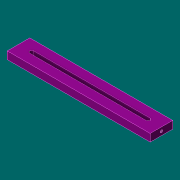
# Autodesk Inventor part: verticalSupourt
Saved by Autodesk Inventor 2016 (Build 200138000, 138)
## iProperties
Created: 2015-10-27
Part Number: verticalSupourt
Material: ABS Plastic
Document SubType Name: Modeling
Designer: Sawaiz
Density: 1.06 g/cm^3
Appearance: Smooth - Purple
Author: Sawaiz
Autodesk Inventor part; units mm, degrees
ref_plane "YZ Plane" through (0, 0, 0) normal (1, 0, 0) x (0, 1, 0)
ref_plane "XZ Plane" through (0, 0, 0) normal (0, 1, 0) x (-1, 0, 0)
ref_plane "XY Plane" through (0, 0, 0) normal (0, 0, 1) x (1, 0, 0)
sketch "Sketch1" plane through (0, 0, 0) normal (0, 0, 1) x (1, 0, 0)
  line L0 (-9.525, -60.325) -> (9.525, -60.325)
  line L1 (9.525, -60.325) -> (9.525, 60.325)
  line L2 (9.525, 60.325) -> (-9.525, 60.325)
  line L3 (-9.525, 60.325) -> (-9.525, -60.325)
  line L4 (-9.525, -60.325) -> (9.525, 60.325) construction
  line L5 (9.525, -60.325) -> (-9.525, 60.325) construction
  point P0 (0, 0)
  dimension "d0" = 19.05
  dimension "d1" = 120.65
  constraints: 12 end point, 2 midpoint, 2 parallel, 1 horizontal, 1 perpendicular
  measures "d0" distance of L2.end L1.end
  measures "d1" distance of L1.end L0.end
extrude "Extrusion1" add sketch "Sketch1" along normal blind 6.35
sketch "Sketch2" plane through (0, 0, 6.35) normal (0, 0, 1) x (1, 0, 0)
  line L0 (1.6891, -50.8) -> (-1.6891, -50.8)
  line L1 (-1.6891, -50.8) -> (-1.6891, 50.8)
  line L2 (-1.6891, 50.8) -> (1.6891, 50.8)
  line L3 (1.6891, 50.8) -> (1.6891, -50.8)
  line L4 (1.6891, -50.8) -> (-1.6891, 50.8) construction
  line L5 (-1.6891, -50.8) -> (1.6891, 50.8) construction
  point P0 (0, 0)
  dimension "d4" = 3.3782
  dimension "d5" = 101.6
  constraints: 12 end point, 2 midpoint, 2 parallel, 1 horizontal, 1 perpendicular
  measures "d4" distance of L1.end L2.end
  measures "d5" distance of L0.end L1.end
extrude "Extrusion2" cut sketch "Sketch2" against normal through all
fillet "Fillet1" radius 1.6891 4 edges at (-1.6891, -50.8, 3.175) (1.6891, -50.8, 3.175) (-1.6891, 50.8, 3.175) (1.6891, 50.8, 3.175)
sketch "Sketch4" plane through (-9.525, -60.325, 0) normal (0, -1, 0) x (1, 0, 0)
  line L0 (0, 0) -> (19.05, 0) projected
  line L1 (19.05, 0) -> (19.05, 6.35) projected
  line L2 (0, 6.35) -> (19.05, 6.35) projected
  line L3 (0, 0) -> (0, 6.35) projected
  point P0 (9.525, 0)
  point P1 (9.525, 3.175)
  dimension "d16" = 3.175
  dimension "d17" = 9.525
  measures "d16" distance from line of L0 point (9.525, 3.175)
  measures "d17" distance from line of L3 point (9.525, 3.175)
hole "Hole2" at (0, -60.325, 3.175) direction (0, 1, 0) diameter 2.156 depth 8.865 tip angle 118 thread size "4-40 UNC" class "2B" standard "ANSI Unified Screw Threads"
mirror "Mirror1" about plane through (0, 0, 0) normal (0, 1, 0) of "Hole2"
equation "\"d0\" = sensorHolderDepth"
equation "\"d1\" = -internalAcrylicThickness + height"
equation "\"d2\" = acrylicThickness"
equation "\"d5\" = height - 4 * acrylicThickness"
equation "\"d6\" = acrylicThickness"
equation "\"d16\" = 0.5 * internalAcrylicThickness"
equation "\"d17\" = 0.5 * sensorHolderDepth"
equation "\"acrylicThickness\" = 6.35"
equation "\"height\" = 127"
equation "\"sensorHolderDepth\" = 19.05"
equation "\"frameAcrylicThickness\" = 9.525"
equation "\"internalAcrylicThicnkess\" = 6.35"
equation "\"width\" = 127"
equation "\"depth\" = 273.05"
equation "\"mirrorAngle\" = 5deg"
equation "\"detectorWidth\" = 52"
equation "\"detectorHeight\" = 52"
equation "\"mirrorThickness\" = 3.175"
equation "\"fresnelThickness\" = 0.1"
equation "\"focalLength\" = 76.2"
equation "\"ior\" = 1.49"
equation "\"centerThickness\" = 1.524"
equation "\"fresnelAngle\" = 90deg"
equation "\"fresnelEffectiveDiameter\" = 152.4"
equation "\"oRingWidth\" = 1.5875"
equation "\"internalAcrylicThickness\" = 6.35"
equation "\"aerogelClearence\" = 3.175"
equation "\"backplaneHoleOffsett\" = 6.35"
equation "\"backplanePCBHeight\" = 76.2"
equation "\"backplanePCBWidth\" = 76.2"
equation "\"backplanePostionOffsett\" = 12.7"
equation "\"moduleSlotClearence\" = 0.79375"
body "Solid1"
